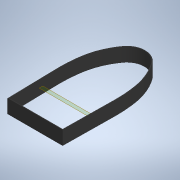
# Autodesk Inventor part: Strap
Saved by Autodesk Inventor 2020 (Build 240168000, 168)
## iProperties
Created: 2019-09-18
Part Number: Strap
Material: Generic
Document SubType Name: Modeling
Designer: suchanek
Density: 1 g/cm^3
Appearance: Default
Author: suchanek
Autodesk Inventor part; units mm, degrees
ref_plane "YZ Plane" through (0, 0, 0) normal (1, 0, 0) x (0, 1, 0)
ref_plane "XZ Plane" through (0, 0, 0) normal (0, 1, 0) x (-1, 0, 0)
ref_plane "XY Plane" through (0, 0, 0) normal (0, 0, 1) x (1, 0, 0)
ref_plane "Work Plane1" through (0, -20, -46.550515) normal (0, -1, 0) x (1, 0, 0)
sketch "Sketch3" plane through (0, 0, 0) normal (1, 0, 0) x (0, 1, 0)
  line L0 (-10, 0.75) -> (-30, 0.75) construction
  line L1 (-10, 1.5) -> (-30, 1.5)
  line L2 (-30, 0) -> (-10, 0)
  arc A0 (-10, 0) -> (-10, 1.5) centre (-10, 0.75) ccw
  arc A1 (-30, 1.5) -> (-30, 0) centre (-30, 0.75) ccw
  line L3 (-20, 0) -> (-20, -75.521339)
  point P0 (0, 0)
  point P1 (-20, 0.75)
  dimension "d0" = 1.5
  dimension "d1" = 20
  constraints: 8 end point, 4 point on circle, 4 tangent, 2 centre point, 2 point on line, 1 horizontal, 1 midpoint, 1 parallel
  measures "d0" diameter of A1
  measures "d1" distance of L1.start L1.end
sketch "Sketch2" plane through (0, -20, -46.550515) normal (0, -1, 0) x (1, 0, 0)
  spline S0 degree 3 poles (10.936352, -107.459737) (7.179934, -102.68902) (4.033535, -97.51867) (-5.225152, -78.100329) (-8.2872, -62.427946) (-10.142521, -35.374288) (-9.704535, -25.423748) (-8.723403, -10.3087) (-7.774117, -1.15603) (-5.538946, 14.831288) (-5.181485, 16.030381) (-4.552811, 20.183892) (-4.390113, 22.146158) (-3.922153, 24.896569) (-3.697268, 25.872669) (-3.076393, 27.34097) (-2.721493, 27.87477) (-1.646581, 28.921839) (-1.096468, 29.286827) (-0.472504, 29.537585) knots -4.25223397 -4.25223397 -4.25223397 -4.25223397 -3.9562506 -3.9562506 -3.20358637 -3.20358637 -2.63296418 -2.63296418 -1.91340599 -1.91340599 -1.25108329 -1.25108329 -0.74740313 -0.74740313 -0.45018243 -0.45018243 -0.20171856 -0.20171856 0 0 0 0
  spline S1 degree 3 poles (-0.472504, 29.537585) (1.662997, 30.394784) (3.76326, 31.18858) (12.066295, 33.674511) (18.105231, 34.719852) (34.355163, 36.098659) (44.970674, 35.327004) (58.349341, 31.895929) (61.353799, 30.795493) (64.451791, 29.553471) knots -7.76000275 -7.76000275 -7.76000275 -7.76000275 -6.95943849 -6.95943849 -5.26298404 -5.26298404 -2.25628604 -2.25628604 -0.98996136 -0.98996136 -0.98996136 -0.98996136
  spline S2 degree 3 poles (64.451791, 29.553471) (64.8398, 29.397595) (65.202558, 29.19622) (65.889779, 28.69381) (66.202675, 28.396571) (67.033071, 27.417933) (67.345172, 26.774592) (68.217927, 24.021686) (68.397755, 21.252198) (68.956077, 17.339933) (69.095411, 16.833196) (70.788197, 6.497314) (71.779174, -1.55009) (73.836501, -23.43642) (74.335881, -37.059566) (71.775195, -64.13545) (69.136912, -76.833848) (61.279747, -95.276855) (57.62611, -101.65135) (53.064616, -107.446458) knots -16.54715867 -16.54715867 -16.54715867 -16.54715867 -16.22687828 -16.22687828 -15.89511657 -15.89511657 -15.24378739 -15.24378739 -13.58830962 -13.58830962 -12.65182165 -12.65182165 -10.37688693 -10.37688693 -6.01428586 -6.01428586 -2.21250171 -2.21250171 0 0 0 0
  line L0 (53.064616, -107.446458) -> (10.936352, -107.459737)
  line L1 (-8, 46.550515) -> (72.7983, 46.550515)
  line L2 (72.7983, 46.550515) -> (72.7983, 36.550515)
  line L3 (72.7983, 36.550515) -> (-8, 36.550515)
  line L4 (-8, 36.550515) -> (-8, 46.550515)
  line L5 (-8, 46.550515) -> (72.7983, 46.550515)
  line L6 (72.7983, 46.550515) -> (72.7983, 36.550515)
  arc A0 (71.065514, -65.184851) -> (73.757347, -30.964682) centre (-115.357252, -33.304478) ccw
  arc A1 (53.064616, -107.446458) -> (71.065514, -65.184851) centre (-26.86172, -48.438202) ccw
  line L7 (-8, 46.550515) -> (-9.732055, -28.970825)
  arc A2 (-9.732055, -28.970825) -> (-7.069542, -65.208874) centre (179.224539, -33.304478) ccw
  arc A3 (-7.069542, -65.208874) -> (10.936352, -107.459737) centre (90.85668, -48.438202) ccw
  arc A4 (10.936352, -107.459737) -> (53.064616, -107.446458) centre (31.995584, -91.907395) ccw
  line L8 (73.757347, -30.964682) -> (72.7983, 46.550515)
  point P0 (0, 46.550515)
  dimension "d2" = 84.98872
  dimension "d7" = 10
  dimension "d8" = 80.7983
  dimension "d9" = 6.99704
  dimension "d10" = 8
  constraints: 18 end point, 10 point on circle, 5 centre point, 5 tangent, 2 horizontal alignment, 1 horizontal, 1 perpendicular, 1 point on line, 1 vertical, 11 other
  measures "d2" distance from line of L3 A1.centre
  measures "d7" distance between parallel lines of L3 L1
  measures "d8" distance of L1.start L1.end
  measures "d9" distance from line of L3 point (64.452, 29.553)
  measures "d10" distance of L1.start point (0, 46.551)
sweep "Sweep1" add profiles "Sketch3" path "Sketch2" path curves A3 A4 A1 A0 L8 L1 L7 A2
body "Solid1"
